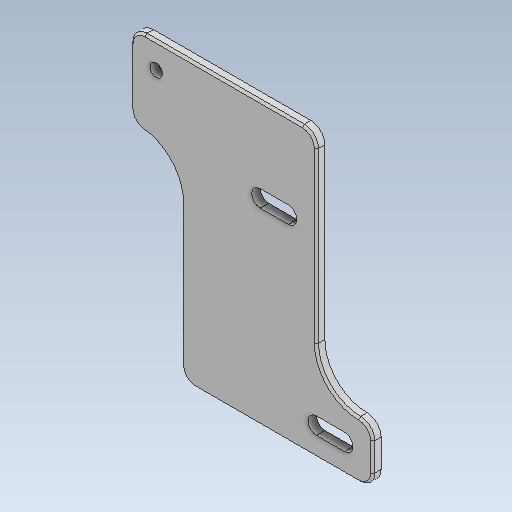
# Autodesk Inventor part: Front
Saved by Autodesk Inventor 2021 (Build 250183000, 183)
## iProperties
Created: 2021-02-16
Part Number: Front
Material: Generic
Document SubType Name: Modeling
Designer: Viktor
Density: 1 g/cm^3
Appearance: Default
Author: Viktor
Autodesk Inventor part; units mm, degrees
ref_plane "YZ Plane" through (0, 0, 0) normal (1, 0, 0) x (0, 1, 0)
ref_plane "XZ Plane" through (0, 0, 0) normal (0, 1, 0) x (-1, 0, 0)
ref_plane "XY Plane" through (0, 0, 0) normal (0, 0, 1) x (1, 0, 0)
sketch "Sketch1" plane through (0, 0, 0) normal (0, 0, 1) x (1, 0, 0)
  line L0 (0, 0) -> (-86, 0)
  line L1 (-86, 0) -> (-86, 100)
  line L2 (-86, 100) -> (-20, 100)
  line L3 (-20, 100) -> (-20, 20)
  line L4 (-20, 20) -> (0, 20)
  line L5 (0, 20) -> (0, 0)
  dimension "d0" = 20
  dimension "d1" = 20
  dimension "d2" = 100
  dimension "d3" = 86
  constraints: 12 end point, 5 perpendicular, 1 horizontal
  measures "d0" distance between parallel lines of L5 L3
  measures "d1" distance of L4.end L0.start
  measures "d2" distance between parallel lines of L0 L2
  measures "d3" distance between parallel lines of L5 L1
extrude "Extrusion1" add sketch "Sketch1" along normal blind 3
sketch "Sketch2" plane through (0, 0, 3) normal (0, 0, 1) x (1, 0, 0)
  line L0 (-86, 0) -> (-68, 0)
  line L1 (-68, 0) -> (-68, 70)
  line L2 (-68, 70) -> (-86, 70)
  line L3 (-86, 70) -> (-86, 0)
  line L4 (-20, 100) -> (-86, 100) projected
  point P0 (0, 0)
  dimension "d6" = 18
  dimension "d7" = 30
  constraints: 8 end point, 2 parallel, 1 horizontal, 1 perpendicular
  measures "d6" distance between parallel lines of L1 L3
  measures "d7" distance between parallel lines of L4 L2
extrude "Extrusion2" cut sketch "Sketch2" against normal blind 3
sketch "Sketch3" plane through (0, 0, 3) normal (0, 0, 1) x (1, 0, 0)
  line L0 (-20, 10) -> (-10, 10) construction
  line L1 (-20, 7) -> (-10, 7)
  line L2 (-10, 13) -> (-20, 13)
  arc A0 (-20, 13) -> (-20, 7) centre (-20, 10) ccw
  arc A1 (-10, 7) -> (-10, 13) centre (-10, 10) ccw
  line L3 (0, 0) -> (0, 20) projected
  line L4 (0, 20) -> (-20, 20) projected
  line L5 (-40, 70) -> (-30, 70) construction
  line L6 (-40, 67) -> (-30, 67)
  line L7 (-30, 73) -> (-40, 73)
  arc A2 (-40, 73) -> (-40, 67) centre (-40, 70) ccw
  arc A3 (-30, 67) -> (-30, 73) centre (-30, 70) ccw
  point P0 (-15, 10)
  point P1 (-35, 70)
  dimension "d10" = 15
  dimension "d11" = 10
  dimension "d12" = 3
  dimension "d13" = 10
  dimension "d14" = 20
  dimension "d15" = 3
  dimension "d16" = 10
  dimension "d17" = 60
  constraints: 16 end point, 8 point on circle, 8 tangent, 4 centre point, 2 midpoint, 2 parallel, 1 horizontal
  measures "d10" distance from line of L3 point (-15, 10)
  measures "d11" distance of L2.start L2.end
  measures "d12" radius of A1
  measures "d13" distance from line of L4 point (-15, 10)
  measures "d14" horizontal distance of point (-35, 70) point (-15, 10)
  measures "d15" radius of A3
  measures "d16" distance of L7.start L7.end
  measures "d17" vertical distance of point (-15, 10) point (-35, 70)
extrude "Extrusion3" cut sketch "Sketch3" against normal blind 3
fillet "Fillet1" radius 5 6 edges at (0, 0, 1.5) (-68, 0, 1.5) (0, 20, 1.5) (-20, 100, 1.5) (-86, 70, 1.5) (-86, 100, 1.5)
fillet "Fillet1" radius 15 2 edges at (-20, 20, 1.5) (-68, 70, 1.5)
sketch "Sketch4" plane through (0, 0, 3) normal (0, 0, 1) x (1, 0, 0)
  circle A0 centre (-77, 91) radius 2.25
  line L0 (-25, 100) -> (-81, 100) projected
  line L1 (-86, 95) -> (-86, 75) projected
  point P0 (0, 0)
  dimension "d22" = 4.5
  dimension "d23" = 9
  dimension "d24" = 9
  constraints: 1 centre point
  measures "d22" diameter of A0
  measures "d23" distance from line of L0 A0.centre
  measures "d24" distance from line of L1 A0.centre
extrude "Extrusion4" cut sketch "Sketch4" against normal blind 3
chamfer "Chamfer1" distance 0.75 angle 45 14 edges at (-71.8757, 65.1626, 3) (-68, 30.0501, 3) (-66.5355, 1.4645, 3) (-34, 0, 3) (-1.4645, 1.4645, 3) (0, 10, 3) (-1.4645, 18.5355, 3) (-15.6066, 24.3934, 3) (-20, 65, 3) (-21.4645, 98.5355, 3) (-53, 100, 3) (-84.5355, 98.5355, 3) (-86, 85, 3) (-84.7081, 71.6459, 3)
equation "\"d15\" = d12"
equation "\"d16\" = d11"
body "Solid1"
